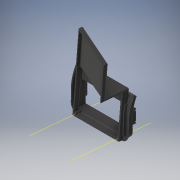
# Autodesk Inventor part: BackPiece_3-7-2018_03
Saved by Autodesk Inventor 2017 (Build 210142000, 142)
## iProperties
Created: 2018-01-24
Part Number: BackPiece_3-7-2018_03
Material: Acetal Resin, Black
Document SubType Name: Modeling
Designer: FadBoard
Density: 1.425 g/cm^3
Appearance: Smooth - Black
Author: FadBoard
Autodesk Inventor part; units mm, degrees
ref_plane "YZ Plane" through (0, 0, 0) normal (1, 0, 0) x (0, 1, 0)
ref_plane "XZ Plane" through (0, 0, 0) normal (0, 1, 0) x (-1, 0, 0)
ref_plane "XY Plane" through (0, 0, 0) normal (0, 0, 1) x (1, 0, 0)
sketch "Sketch1" plane through (0, 0, 0) normal (0, 0, 1) x (1, 0, 0)
  line L0 (-86.36, -50.038) -> (86.36, -50.038)
  line L1 (88.9, -47.498) -> (88.9, 47.498)
  line L2 (86.36, 50.038) -> (-86.36, 50.038)
  line L3 (-88.9, 47.498) -> (-88.9, -47.498)
  line L4 (-88.9, -50.038) -> (88.9, 50.038) construction
  line L5 (88.9, -50.038) -> (-88.9, 50.038) construction
  arc A0 (-86.36, 50.038) -> (-88.9, 47.498) centre (-86.36, 47.498) ccw
  arc A1 (-88.9, -47.498) -> (-86.36, -50.038) centre (-86.36, -47.498) ccw
  arc A2 (86.36, -50.038) -> (88.9, -47.498) centre (86.36, -47.498) ccw
  arc A3 (88.9, 47.498) -> (86.36, 50.038) centre (86.36, 47.498) ccw
  point P0 (0, 0)
  dimension "d0" = 177.8
  dimension "d1" = 100.076
  dimension "d2" = 2.54
  dimension "d24" = 100.076
  dimension "d25" = 177.8
  constraints: 12 end point, 8 point on circle, 8 point on line, 8 tangent, 4 centre point, 3 equal radius, 2 midpoint, 2 parallel, 1 horizontal, 1 perpendicular
  measures "d0" distance of L5.end L4.end
  measures "d1" distance of L4.end L5.start
  measures "d2" radius of A0
  measures "d24" distance between parallel lines of L0 L2
  measures "d25" distance between parallel lines of L3 L1
extrude "Extrusion1" add sketch "Sketch1" along normal blind 17.78
sketch "Sketch3" plane through (0, 0, 0) normal (1, 0, 0) x (0, 1, 0)
  line L0 (-63.8556, 32.1039) -> (79.9846, 32.1039)
  line L1 (-56.2356, 17.6259) -> (16.2941, 17.6259)
  arc A0 (74.8157, 2.8177) -> (16.2941, 17.6259) centre (10.1563, -129.6725) ccw
  arc A1 (-56.2356, 17.6259) -> (-63.8556, 32.1039) centre (-75.5729, 16.6927) ccw
  line L2 (74.8157, 2.8177) -> (79.9846, 10.5247)
  line L3 (79.9846, 32.1039) -> (79.9846, 10.5247)
  point P0 (0, 0)
  dimension "d21" = 143.8402
  constraints: 8 end point, 4 point on circle, 2 centre point, 1 horizontal
  measures "d21" distance of L0.start L0.end
extrude "Extrusion3" add sketch "Sketch3" along normal mid plane 212.09
sketch "Sketch7" plane through (0, 0, 0) normal (0, 0, -1) x (-1, 0, 0)
  line L0 (-83.82, -44.958) -> (83.82, -44.958)
  line L1 (83.82, -44.958) -> (83.82, 44.958)
  line L2 (83.82, 44.958) -> (-83.82, 44.958)
  line L3 (-83.82, 44.958) -> (-83.82, -44.958)
  line L4 (-86.36, -50.038) -> (86.36, -50.038) projected
  line L5 (86.36, 50.038) -> (-86.36, 50.038) projected
  line L6 (-88.9, 47.498) -> (-88.9, -47.498) projected
  line L7 (88.9, -47.498) -> (88.9, 47.498) projected
  point P0 (0, 0)
  dimension "d33" = 5.08
  dimension "d34" = 5.08
  dimension "d35" = 5.08
  dimension "d36" = 5.08
  constraints: 8 end point, 2 parallel, 1 horizontal, 1 perpendicular
  measures "d33" distance between parallel lines of L4 L0
  measures "d34" distance between parallel lines of L2 L5
  measures "d35" distance between parallel lines of L3 L6
  measures "d36" distance between parallel lines of L7 L1
extrude "Extrusion5" cut sketch "Sketch7" against normal up to next
fillet "Fillet1" radius 23.368 2 edges at (-106.045, -58.4411, 25.7094) (106.045, -58.4411, 25.7094)
shell "Shell1" thickness 3.81 removed faces 1 at (-27.94, 68.309, 32.1039)
sketch "Sketch11" plane through (0, 0, 0) normal (0, 0, -1) x (-1, 0, 0)
  line L0 (-83.82, 44.958) -> (-83.82, -44.958) projected
  line L1 (83.82, 44.958) -> (83.82, -44.958) projected
  line L2 (-93.345, 24.003) -> (-86.995, 24.003)
  line L3 (-86.995, 24.003) -> (-86.995, -24.0538)
  line L4 (-86.995, -24.0538) -> (-93.345, -24.0538)
  line L5 (-93.345, -24.0538) -> (-93.345, 24.003)
  line L6 (-83.82, 44.958) -> (83.82, 44.958) projected
  line L7 (86.995, 24.003) -> (93.345, 24.003)
  line L8 (93.345, 24.003) -> (93.345, -24.0538)
  line L9 (93.345, -24.0538) -> (86.995, -24.0538)
  line L10 (86.995, -24.0538) -> (86.995, 24.003)
  point P0 (0, 0)
  dimension "d303" = 6.35
  dimension "d304" = 48.0568
  dimension "d306" = 20.955
  dimension "d307" = 3.175
  dimension "d308" = 6.35
  dimension "d309" = 48.0568
  dimension "d310" = 20.955
  dimension "d311" = 3.175
  constraints: 16 end point, 4 parallel, 2 horizontal, 2 perpendicular
  measures "d303" distance of L3.end L4.end
  measures "d304" distance of L2.end L3.end
  measures "d306" distance between parallel lines of L6 L2
  measures "d307" distance between parallel lines of L0 L3
  measures "d308" distance of L8.end L9.end
  measures "d309" distance of L7.end L8.end
  measures "d310" distance between parallel lines of L7 L6
  measures "d311" distance between parallel lines of L10 L1
extrude "Extrusion9" add sketch "Sketch11" along normal blind 8.89 and the other way blind 10.795
chamfer "Chamfer1" distance 1.27 angle 45 20 edges at (0, 50.038, 0) (88.1561, 49.2941, 0) (88.9, 35.7505, 0) (-88.1561, 49.2941, 0) (-88.9, 35.7505, 0) (88.9, -35.7759, 0) (88.1561, -49.2941, 0) (0, -50.038, 0) (-88.1561, -49.2941, 0) (-88.9, -35.7759, 0) (-93.345, 24.003, 0.9525) (-93.345, -0.0254, -8.89) (-93.345, -24.0538, 0.9525) (-90.17, 24.003, -8.89) (-90.17, -24.0538, -8.89) (90.17, 24.003, -8.89) (93.345, 24.003, 0.9525) (90.17, -24.0538, -8.89) (93.345, -0.0254, -8.89) (93.345, -24.0538, 0.9525)
sketch "Sketch12" plane through (88.9, -47.498, 17.6259) normal (1, 0, 0) x (0, 0, -1)
  line L0 (20.3564, 28.9751) -> (22.8075, 28.9751) construction
  line L1 (20.3564, 27.4511) -> (22.8075, 27.4511)
  line L2 (22.8075, 30.4991) -> (20.3564, 30.4991)
  arc A0 (20.3564, 30.4991) -> (20.3564, 27.4511) centre (20.3564, 28.9751) ccw
  arc A1 (22.8075, 27.4511) -> (22.8075, 30.4991) centre (22.8075, 28.9751) ccw
  line L3 (20.3564, 65.132) -> (22.8075, 65.132) construction
  line L4 (20.3564, 63.608) -> (22.8075, 63.6079)
  line L5 (22.8075, 66.656) -> (20.3564, 66.656)
  arc A2 (20.3564, 66.656) -> (20.3564, 63.608) centre (20.3564, 65.132) ccw
  arc A3 (22.8075, 63.6079) -> (22.8075, 66.656) centre (22.8075, 65.132) ccw
  point P0 (21.582, 28.9751)
  point P1 (21.582, 65.132)
  dimension "d99" = 3.048
  dimension "d100" = 5.4991
  dimension "d101" = 3.048
  dimension "d102" = 5.4991
  dimension "d103" = 36.1569
  constraints: 16 end point, 8 point on circle, 8 tangent, 4 centre point, 2 horizontal, 2 midpoint, 2 parallel
  measures "d99" diameter of A1
  measures "d101" diameter of A3
  measures "d103" distance of point (21.582, 28.975) point (21.582, 65.132)
extrude "Extrusion10" cut sketch "Sketch12" along normal through all both and the other way through all
sketch "Sketch13" plane through (88.9, -47.498, 17.6259) normal (1, 0, 0) x (0, 0, -1)
  line L0 (20.9914, 28.9751) -> (26.0714, 28.9751) construction
  line L1 (20.9914, 25.8001) -> (26.0714, 25.8001)
  line L2 (26.0714, 32.1501) -> (20.9914, 32.1501)
  arc A0 (20.9914, 32.1501) -> (20.9914, 25.8001) centre (20.9914, 28.9751) ccw
  arc A1 (26.0714, 25.8001) -> (26.0714, 32.1501) centre (26.0714, 28.9751) ccw
  line L3 (20.3564, 65.132) -> (25.4364, 65.132) construction
  line L4 (20.3564, 61.957) -> (25.4364, 61.957)
  line L5 (25.4364, 68.307) -> (20.3564, 68.307)
  arc A2 (20.3564, 68.307) -> (20.3564, 61.957) centre (20.3564, 65.132) ccw
  arc A3 (25.4364, 61.957) -> (25.4364, 68.307) centre (25.4364, 65.132) ccw
  line L6 (26.5159, 23.4569) -> (26.5159, 71.501) projected
  line L7 (17.6259, 23.4569) -> (26.5159, 23.4569) projected
  point P0 (17.6259, 47.498)
  point P1 (23.5314, 28.9751)
  point P2 (22.8964, 65.132)
  dimension "d109" = 6.35
  dimension "d110" = 11.43
  dimension "d111" = 6.35
  dimension "d112" = 11.43
  dimension "d113" = 36.1569
  dimension "d121" = 6.1595
  dimension "d123" = 5.5182
  constraints: 16 end point, 8 point on circle, 8 tangent, 4 centre point, 2 horizontal, 2 midpoint, 2 parallel
  measures "d109" diameter of A1
  measures "d111" diameter of A3
  measures "d113" vertical distance of point (23.531, 28.975) point (22.896, 65.132)
  measures "d121" distance from line of L6 L3.start
  measures "d123" distance from line of L7 point (23.531, 28.975)
extrude "Extrusion11" cut sketch "Sketch13" along normal blind 6.35
sketch "Sketch14" plane through (-88.9, -47.498, 17.6259) normal (-1, 0, 0) x (0, 0, 1)
  line L0 (-25.7934, 28.9751) -> (-20.7134, 28.9751) construction
  line L1 (-25.7934, 25.8001) -> (-20.7134, 25.8001)
  line L2 (-20.7134, 32.1501) -> (-25.7934, 32.1501)
  arc A0 (-25.7934, 32.1501) -> (-25.7934, 25.8001) centre (-25.7934, 28.9751) ccw
  arc A1 (-20.7134, 25.8001) -> (-20.7134, 32.1501) centre (-20.7134, 28.9751) ccw
  line L3 (-25.4364, 65.132) -> (-20.3564, 65.132) construction
  line L4 (-25.4364, 61.957) -> (-20.3564, 61.957)
  line L5 (-20.3564, 68.307) -> (-25.4364, 68.307)
  arc A2 (-25.4364, 68.307) -> (-25.4364, 61.957) centre (-25.4364, 65.132) ccw
  arc A3 (-20.3564, 61.957) -> (-20.3564, 68.307) centre (-20.3564, 65.132) ccw
  line L6 (-26.5159, 71.501) -> (-26.5159, 23.4569) projected
  line L7 (-26.5159, 23.4569) -> (-17.6259, 23.4569) projected
  point P0 (-17.6259, 47.498)
  point P1 (-28.5239, 47.9916)
  point P2 (-23.2534, 28.9751)
  point P3 (-22.8964, 65.132)
  dimension "d116" = 6.35
  dimension "d117" = 11.43
  dimension "d118" = 6.35
  dimension "d119" = 11.43
  dimension "d120" = 36.1569
  dimension "d122" = 6.1595
  dimension "d124" = 5.5182
  constraints: 16 end point, 8 point on circle, 8 tangent, 4 centre point, 2 horizontal, 2 midpoint, 2 parallel
  measures "d116" diameter of A1
  measures "d118" diameter of A3
  measures "d120" vertical distance of point (-23.253, 28.975) point (-22.896, 65.132)
  measures "d122" distance from line of L6 L3.end
  measures "d124" distance between parallel lines of L7 L0
extrude "Extrusion12" cut sketch "Sketch14" along normal blind 6.35
fillet "Fillet2" radius 6.35 2 edges at (-106.045, 79.9846, 21.3143) (106.045, 79.9846, 21.3143)
sketch "Sketch15" plane through (0, 0, 0) normal (1, 0, 0) x (0, 1, 0)
  line L0 (-63.8556, 32.1039) -> (48.768, 22.3712)
  line L1 (203.0053, 0.7169) -> (205.0209, 24.0399)
  line L2 (-62.5542, 47.1632) -> (-63.8556, 32.1039)
  line L3 (76.1746, 11.684) -> (73.481, 7.6679)
  line L4 (73.481, 7.6679) -> (48.768, 16.5518)
  line L5 (76.1703, 11.6777) -> (203.0053, 0.7169)
  line L6 (48.768, 22.3712) -> (48.768, 16.5518)
  line L7 (90.4582, 33.9401) -> (99.8787, 142.9505)
  line L8 (213.4949, 122.098) -> (205.0209, 24.0399)
  line L9 (90.4582, 33.9401) -> (-62.5542, 47.1632)
  line L10 (99.8787, 142.9505) -> (213.4949, 122.098)
  point P0 (0, 0)
  constraints: 22 end point, 4 perpendicular, 1 point on line, 1 vertical
extrude "Extrusion13" add sketch "Sketch15" along normal mid plane 170.18
sketch "Sketch16" plane through (-85.09, -62.5542, 47.1632) normal (0, 0.0860972, 0.9962867) x (1, 0, 0)
  line L0 (3.81, 261.112) -> (166.37, 261.112)
  line L1 (166.37, 261.112) -> (166.37, 3.81)
  line L2 (166.37, 3.81) -> (3.81, 3.81)
  line L3 (3.81, 3.81) -> (3.81, 261.112)
  line L4 (0, 264.922) -> (170.18, 264.922) projected
  line L5 (0, 0) -> (0, 264.922) projected
  line L6 (170.18, 264.922) -> (170.18, 0) projected
  line L7 (0, 0) -> (170.18, 0) projected
  point P0 (85.09, 66.3826)
  dimension "d210" = 3.81
  dimension "d211" = 3.81
  dimension "d212" = 3.81
  dimension "d213" = 3.81
  dimension "d214" = 257.302
  dimension "d215" = 162.56
  constraints: 8 end point, 2 parallel, 1 horizontal, 1 perpendicular
  measures "d210" distance between parallel lines of L0 L4
  measures "d211" distance between parallel lines of L5 L3
  measures "d212" distance between parallel lines of L1 L6
  measures "d213" distance from line of L1.end L7
  measures "d214" distance between parallel lines of L0 L2
  measures "d215" distance between parallel lines of L1 L3
extrude "Extrusion14" [suppressed]
fillet "Fillet3" [suppressed]
sketch "Sketch18" plane through (-85.09, -63.6477, 34.5103) normal (0, 0.0860972, 0.9962867) x (1, 0, 0)
  line L0 (0, 112.5911) -> (170.18, 112.5911)
  line L1 (170.18, 112.5911) -> (170.18, 14.8957)
  line L2 (170.18, 14.8957) -> (0, 14.8957)
  line L3 (0, 14.8957) -> (0, 112.5911)
  point P0 (85.09, 66.3826)
  constraints: 8 end point, 2 parallel, 1 horizontal, 1 perpendicular
extrude "Extrusion16" [suppressed]
sketch "Sketch19" plane through (-106.045, 0, 0) normal (-1, 0, 0) x (0, 0, 1)
  line L0 (50.1715, -65.5208) -> (41.3, 85.6042)
  line L1 (32.2093, -65.5208) -> (31.1124, 17.2348)
  arc A0 (31.1124, 17.2348) -> (9.5545, 82.2323) centre (-115.7707, 4.5915) ccw
  line L2 (9.5545, 82.2323) -> (19.7207, 85.6042)
  line L3 (41.3, 85.6042) -> (19.7207, 85.6042)
  line L4 (32.2093, -65.5208) -> (50.1715, -65.5208)
  line L5 (32.1039, 73.6346) -> (3.3876, 73.6346) projected
  line L6 (32.1039, 79.9846) -> (32.1039, 73.6346) projected
  point P0 (0, 0)
  point P1 (9.196, 5.6196)
  dimension "d167" = 8.5978
  dimension "d168" = 22.5494
  constraints: 10 end point, 2 point on circle, 1 centre point, 1 horizontal
  measures "d167" distance from line of L2.start L5
  measures "d168" distance from line of L2.start L6
extrude "Extrusion17" cut sketch "Sketch19" against normal up to surface (20.955 mm away)
sketch "Sketch20" plane through (106.045, 0, 0) normal (1, 0, 0) x (0, 0, -1)
  line L0 (-50.2719, -65.5208) -> (-41.4003, 85.6042)
  line L1 (-32.3097, -65.5208) -> (-31.2128, 17.2348)
  arc A0 (-9.5545, 82.2323) -> (-31.2128, 17.2348) centre (115.654, 4.4035) ccw
  line L2 (-9.5545, 82.2323) -> (-19.8211, 85.6042)
  line L3 (-41.4003, 85.6042) -> (-19.8211, 85.6042)
  line L4 (-32.3097, -65.5208) -> (-50.2719, -65.5208)
  line L5 (-32.1039, 73.6346) -> (-3.3876, 73.6346) projected
  line L6 (-32.1039, 73.6346) -> (-32.1039, -35.7212) projected
  point P0 (0, 0)
  point P1 (-13.0745, 0.7401)
  point P2 (-9.2906, 6.3597)
  dimension "d166" = 8.5978
  dimension "d169" = 22.5494
  constraints: 10 end point, 2 point on circle, 1 centre point
  measures "d166" distance from line of L5 L2.start
  measures "d169" distance from line of L6 L2.start
extrude "Extrusion18" cut sketch "Sketch20" against normal up to surface (20.955 mm away)
sketch "Sketch21" plane through (83.82, 44.958, 17.6259) normal (0, 0, -1) x (-1, 0, 0)
  line L0 (0, -89.916) -> (0, 0) projected
  line L1 (167.64, 0) -> (165.1, 0) projected
  line L2 (0, -89.916) -> (167.64, -89.916)
  line L3 (167.64, -89.916) -> (167.64, 0)
  line L4 (167.64, 0) -> (0, 0)
  line L5 (0, 0) -> (0, -89.916)
  point P0 (83.82, -44.958)
  point P1 (0, -68.9991)
  dimension "d321" = 167.64
  constraints: 8 end point, 2 parallel, 1 horizontal, 1 perpendicular
  measures "d321" distance between parallel lines of L3 L0
extrude "Extrusion19" [suppressed]
ref_plane "Work Plane1" through (0, 24.003, 0) normal (1, 0, 0) x (0, 0, -1)
sketch "Sketch22" plane through (0, 24.003, 0) normal (1, 0, 0) x (0, 0, -1)
  line L0 (-0.7169, 179.0023) -> (-11.3481, 55.9816) projected
  line L1 (-21.5221, 26.0559) -> (8.4661, 26.0559)
  line L2 (-1.27, 26.035) -> (-12.2569, 26.035) projected
  line L3 (8.4661, 26.0559) -> (8.4661, 45.9608)
  line L4 (8.4661, 45.9608) -> (-19.0412, 45.9608)
  line L5 (-19.0412, 45.9608) -> (-21.5221, 26.0559)
  point P0 (0, -24.003)
  point P1 (-0.9902, 175.8391)
  point P2 (0, 26.035)
  constraints: 8 end point, 2 perpendicular, 1 parallel
extrude "Extrusion20" cut sketch "Sketch22" along normal mid plane 152.4
ref_plane "Work Plane5" through (-78.9713, 89.3285, 20.8673) normal (-0.4226183, 0.0780306, 0.9029424) x (0, 0.9962867, -0.0860972)
ref_plane "Work Plane4" through (-85.09, 90.4582, 33.9401) normal (-0.4226183, 0.0780306, 0.9029424) x (0, 0.9962867, -0.0860972)
sketch "Sketch33" plane through (-78.9713, 89.3285, 20.8673) normal (-0.4226183, 0.0780306, 0.9029424) x (0, 0.9962867, -0.0860972)
  line L0 (190.9519, -236.9461) -> (4.1858, -236.9461)
  line L1 (4.1858, -236.9461) -> (4.1858, 45.6235)
  line L2 (4.1858, 45.6235) -> (190.9519, 45.6235)
  line L3 (190.9519, 45.6235) -> (190.9519, -236.9461)
  point P0 (-87.2002, -59.5358)
  constraints: 8 end point, 2 parallel, 1 horizontal, 1 perpendicular
extrude "Extrusion32" cut sketch "Sketch33" against normal blind 104.775
sketch "Sketch34" plane through (-85.09, 90.4582, 33.9401) normal (-0.4226183, 0.0780306, 0.9029424) x (0, 0.9962867, -0.0860972)
  line L0 (145.9468, 9.3801) -> (-8.4463, 9.3801)
  line L1 (-8.4463, 9.3801) -> (-8.4463, -215.5316)
  line L2 (-8.4463, -215.5316) -> (145.9468, -215.5316)
  line L3 (145.9468, -215.5316) -> (145.9468, 9.3801)
  point P0 (-87.2002, -59.5358)
  constraints: 8 end point, 2 parallel, 1 horizontal, 1 perpendicular
extrude "Extrusion33" cut sketch "Sketch34" along normal blind 104.775
ref_plane "Work Plane6" through (-81.915, 199.9771, 9.9275) normal (0, 0.9962867, -0.0860972) x (0.9063078, 0.0363862, 0.421049)
sketch "Sketch35" plane through (-81.915, 199.9771, 9.9275) normal (0, 0.9962867, -0.0860972) x (0.9063078, 0.0363862, 0.421049)
  line L0 (2.4773, -3.81) -> (10.6681, -21.3754)
  line L1 (6.7512, -14.478) -> (0, 0) projected
  line L2 (10.6681, -21.3754) -> (188.7291, -18.5785)
  line L3 (188.7291, -18.5785) -> (181.8424, -3.81)
  line L4 (181.8424, -3.81) -> (2.4773, -3.81)
  line L5 (184.2696, 0) -> (-3.5032, 0) projected
  point P0 (62.7838, 59.1871)
  point P1 (3.248, -14.478)
  point P2 (191.0208, -14.478)
  point P3 (180.7664, 0)
  dimension "d465" = 3.81
  dimension "d466" = 3.81
  dimension "d467" = 3.81
  constraints: 8 end point, 2 parallel, 1 horizontal
  measures "d465" distance from line of point (3.248, -14.478) L0
  measures "d466" distance from line of point (191.021, -14.478) L3
  measures "d467" distance between parallel lines of L5 L4
extrude "Extrusion34" cut sketch "Sketch35" against normal blind 112.7125
sketch "Sketch36" plane through (-81.915, -62.5542, 47.1632) normal (0, 0.0860972, 0.9962867) x (1, 0, 0)
  line L0 (0.635, 153.5827) -> (0.635, 264.7624) projected
  line L1 (0.635, 153.5827) -> (163.195, 153.5827)
  line L2 (163.195, 153.5827) -> (163.195, 9.4806)
  line L3 (163.195, 9.4806) -> (0.635, 9.4806)
  line L4 (0.635, 9.4806) -> (0.635, 153.5827)
  line L5 (167.005, 153.5827) -> (167.005, 0) projected
  line L6 (-3.175, 0) -> (167.005, 0) projected
  point P0 (81.915, 66.3826)
  point P1 (167.005, 3.175)
  point P2 (0, 0)
  point P3 (163.83, 0)
  dimension "d470" = 3.81
  constraints: 8 end point, 2 parallel, 1 horizontal, 1 perpendicular, 1 point on line
  measures "d470" distance between parallel lines of L5 L2
extrude "Extrusion35" cut sketch "Sketch36" against normal blind 19.6088 draft -5
sketch "Sketch37" plane through (-81.915, -64.2425, 27.6272) normal (0, 0.0860972, 0.9962867) x (1, 0, 0)
  line L0 (3.9299, 136.3514) -> (159.1923, 136.3514)
  line L1 (159.1923, 136.3514) -> (159.1923, 113.8984)
  line L2 (159.1923, 113.8984) -> (3.9299, 113.8984)
  line L3 (3.9299, 113.8984) -> (3.9299, 136.3514)
  point P0 (81.915, 66.3826)
  constraints: 8 end point, 2 parallel, 1 horizontal, 1 perpendicular
extrude "Extrusion36" add sketch "Sketch37" against normal blind 3.81
fillet "Fillet13" radius 3.81 3 edges at (0, 207.0619, 47.6575) (-85.09, 148.4495, 12.8966) (85.09, 155.2818, 91.9582)
fillet "Fillet14" radius 3.81 4 edges at (85.09, 100.1901, 97.9373) (85.09, 96.3492, 53.4924) (-85.09, 93.5107, 20.6457) (-85.09, 92.9331, 13.9617)
sketch "Sketch38" plane through (-85.09, 0, 0) normal (-1, 0, 0) x (0, 0, 1)
  line L0 (51.9077, -69.6917) -> (32.0924, -69.6917)
  line L1 (32.0924, -69.6917) -> (32.0924, -60.5771)
  line L2 (32.0924, -60.5771) -> (51.9077, -58.1786)
  line L3 (51.9077, -58.1786) -> (51.9077, -69.6917)
  point P0 (0, 0)
  constraints: 8 end point, 1 horizontal, 1 parallel, 1 perpendicular
extrude "Extrusion37" cut sketch "Sketch38" against normal through all
sketch "Sketch39" plane through (-81.28, -53.1088, 46.3469) normal (0, 0.0860972, 0.9962867) x (1, 0, 0)
  circle A0 centre (3.048, -0.547) radius 5.08
  line L0 (-3.81, -5.7046) -> (-3.81, 144.1021) projected
  circle A1 centre (159.512, -0.547) radius 5.08
  line L1 (166.37, 144.1021) -> (166.37, -5.7046) projected
  line L2 (-3.81, -5.7046) -> (166.37, -5.7046) projected
  point P0 (81.28, 56.902)
  point P1 (166.37, 259.0918)
  point P2 (-3.81, 259.0918)
  dimension "d483" = 10.16
  dimension "d529" = 6.858
  dimension "d530" = 10.16
  dimension "d531" = 6.858
  dimension "d543" = 259.6388
  dimension "d544" = 259.6388
  constraints: 2 centre point
  measures "d483" diameter of A0
  measures "d529" distance from line of A0.centre L0
  measures "d530" diameter of A1
  measures "d531" distance from line of L1 A1.centre
  measures "d543" vertical distance of point (166.37, 259.092) A1.centre
  measures "d544" vertical distance of A0.centre point (-3.81, 259.092)
extrude "Extrusion38" add sketch "Sketch39" against normal through all
ref_plane "Work Plane7" through (86.36, -50.038, 17.3719) normal (0, 0, -1) x (-1, 0, 0)
hole "Hole12" at (-78.232, -56.1619, 17.3719) direction (0, 0.0860972, 0.9962867) diameter 3.175 end through all counterbore diameter 7.62 counterbore depth 8.89
hole "Hole13" at (78.232, -56.1619, 17.3719) direction (0, 0.0860972, 0.9962867) diameter 3.175 end through all counterbore diameter 7.62 counterbore depth 8.89
body "Solid1"
